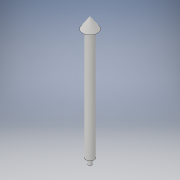
# Autodesk Inventor part: xyz_Axis_with_ball_Axis
Saved by Autodesk Inventor 2018.2 (Build 222227000, 227)
## iProperties
Created: 2018-06-07
Part Number: xyz_Axis_with_ball_Axis
Material: Generisch
Document SubType Name: Modeling
Designer: Nick Koch
Density: 1 g/cm^3
Appearance: Vorgabe
Author: Nick Koch
Autodesk Inventor part; units mm, degrees
ref_plane "Arbeitsebene1" through (0, 0, 0) normal (-1, 0, 0) x (0, -1, 0)
ref_plane "Arbeitsebene7" through (0, 0, 2.2393) normal (0, 0, 1) x (1, 0, 0)
sketch "Skizze6" plane through (0, 0, 2.2393) normal (0, 0, 1) x (1, 0, 0)
  circle A0 centre (0, 0) radius 1.1115
  constraints: 1 centre point, 1 coincident
extrude "Extrusion6" add sketch "Skizze6" along normal blind 30
ref_plane "Arbeitsebene10" through (0, 0, 32.2393) normal (-1, 0, 0) x (0, 0, 1)
sketch "Skizze8" plane through (0, 0, 32.2393) normal (-1, 0, 0) x (0, 0, 1)
  line L0 (0, 0) -> (3, 0)
  line L1 (0, 0) -> (0, 2)
  line L2 (0, 2) -> (3, 0)
  line L3 (-42.2872, 0) -> (10.5479, 0) projected
  point P0 (-32.2393, 0)
  dimension "d17" = 3
  dimension "d18" = 2
  constraints: 6 end point, 1 horizontal, 1 vertical
  measures "d17" distance of L0.start L0.end
  measures "d18" distance of L0.start L1.end
revolve "Umdrehung2" add sketch "Skizze8" angle 360 about axis through (0, 0, 32.2393) along (0, 0, 1)
sketch "Skizze11" plane through (0, 0, 2.2393) normal (0, 0, -1) x (-1, 0, 0)
  circle A0 centre (0, 0) radius 0.5
  dimension "d26" = 1
  constraints: 1 centre point, 1 coincident
  measures "d26" diameter of A0
extrude "Extrusion7" add sketch "Skizze11" along normal blind 1.5
